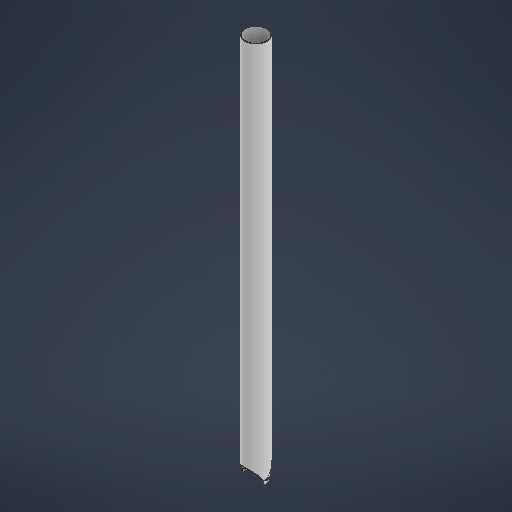
# Autodesk Inventor part: Output link body_ final
Saved by Autodesk Inventor 2026.3 (Build 303398000, 398)
## iProperties
Created: 2026-07-24
Part Number: Output link body_ final
Material: Generic
Document SubType Name: Sheet Metal
Designer: matot
Density: 1 g/cm^3
Sheet Metal Rule: Default_mm
Appearance: Default
Author: matot
Autodesk Inventor part; units mm, degrees
ref_plane "YZ Plane" through (0, 0, 0) normal (1, 0, 0) x (0, 1, 0)
sketch "Sketch1" plane through (0, 0, 0) normal (0, 1, 0) x (-1, 0, 0)
  circle A0 centre (0, 0) radius 15.875
  dimension "d0" = 31.75
  constraints: 1 centre point, 1 coincident
  measures "d0" diameter of A0
extrude "Extrusion1" add sketch "Sketch1" along normal blind 550
sketch "Sketch7" plane through (0, 550, 0) normal (0, 1, 0) x (1, 0, 0)
  circle A0 centre (0, 0) radius 15.075
  dimension "d23" = 30.15
  constraints: 1 centre point, 1 coincident
  measures "d23" diameter of A0
extrude "Extrusion3" cut sketch "Sketch7" against normal through all
sketch "Sketch8" plane through (0, 0, 0) normal (0, -1, 0) x (1, 0, 0)
  circle A0 centre (0, 0) radius 15.875 projected
  point P0 (0, 15.875)
  constraints: 1 vertical alignment, 1 other
ref_plane "Work Plane3" through (0, 0, 15.875) normal (0, 0, 1) x (1, 0, 0)
sketch "Sketch9" plane through (0, 0, 15.875) normal (0, 0, 1) x (1, 0, 0)
  arc A0 (15.075, 5) -> (-15.075, 5) centre (0, 5) ccw
  line L0 (-15.075, 5) -> (-15.075, 0)
  line L1 (15.875, 0) -> (-15.875, 0) projected
  line L2 (15.075, 5) -> (15.075, 0)
  point P0 (0, 0)
  dimension "d26" = 5
  dimension "d27" = 30.15
  constraints: 4 end point, 2 point on circle, 2 point on line, 1 centre point, 1 parallel, 1 tangent, 1 vertical
  measures "d26" distance of point (0, 0) A0.centre
  measures "d27" diameter of A0
extrude "Extrusion4" cut sketch "Sketch9" against normal through all
sketch "Sketch10" plane through (0, 0, 0) normal (0, -1, 0) x (1, 0, 0)
  circle A0 centre (0, 0) radius 15.875 projected
  point P0 (15.875, 0)
  constraints: 1 horizontal alignment, 1 other
ref_plane "Work Plane4" through (15.875, 0, 0) normal (1, 0, 0) x (0, 1, 0)
sketch "Sketch11" plane through (15.875, 0, 0) normal (1, 0, 0) x (0, 1, 0)
  line L0 (0, -4.9759) -> (0, 4.9759) projected
  point P0 (0, 0)
  point P1 (5, 0)
  point P2 (0, 0)
  dimension "d30" = 5
  constraints: 1 midpoint
  measures "d30" distance of point (0, 0) point (5, 0)
hole "Hole3" at (15.875, 5, 0) direction (-1, 0, 0) diameter 3.4587 end through all thread size "M4x0.5" class "6H" standard "ISO Metric profile"
equation "\"d36\" = Thickness"
equation "\"BendRadius\" = Thickness"
equation "\"BendReliefWidth\" = Thickness"
equation "\"BendReliefDepth\" = 0.5 * Thickness"
equation "\"CornerReliefSize\" = 4 * Thickness"
equation "\"MinimumRemnant\" = 2 * Thickness"
equation "\"TransitionRadius\" = BendRadius"
equation "\"JacobiRadiusSize\" = BendRadius"
equation "\"GapSize\" = Thickness"
equation "\"Thickness\" = 0.5"
body "Solid1"
